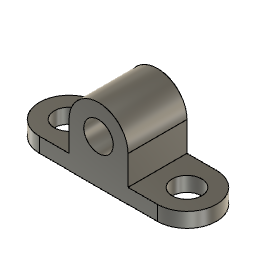
A4 v0 (Autodesk Fusion 360 design; units mm, degrees)
Autodesk Fusion 360 part; units mm, degrees
sketch "Sketch1" plane through (0, 0, 0) normal (0, 0, 1) x (1, 0, 0)
  line L0 (40, -20) -> (-40, -20)
  line L1 (-40, 20) -> (40, 20)
  circle A0 centre (40, 0) radius 10
  circle A1 centre (-40, 0) radius 10
  arc A2 (24, -12) -> (40, 20) centre (40, 0) ccw
  arc A3 (-40, 20) -> (-40, -20) centre (-40, 0) ccw
  dimension "d1" = 80
  dimension "d2" = 40
  dimension "d5" = 40
  dimension "d6" = 40
  constraint horizontal L0
  constraint parallel L0 L1
  measures "d1" distance of L1.start L1.end
  measures "d2" distance of L0.end L1.start
  measures "d5" diameter of A2
  measures "d6" diameter of A3
extrude "Extrude1" add sketch "Sketch1" along normal blind 10
sketch "Sketch2" plane through (0, 0, 0) normal (0, 1, 0) x (1, 0, 0)
  line L0 (-20, 0.1287) -> (20, 0.1287)
  line L1 (20, 0.1287) -> (20, -29.8713)
  line L2 (-20, -29.8713) -> (-20, 0.1287)
  line L3 (-40, 0) -> (-40, -10)
  circle A0 centre (0, -29.8713) radius 10
  arc A1 (-20, -29.8713) -> (20, -29.8713) centre (0, -29.8713) ccw
  dimension "d12" = 40
  dimension "d13" = 30
  dimension "d14" = 20
  dimension "d15" = 20
  dimension "d16" = 20
  constraint horizontal L0
  constraint vertical L1
  constraint vertical L2
  constraint concentric A0 A1
  measures "d12" distance of L0.start L0.end
  measures "d13" distance of L0.start L2.start
  measures "d14" distance of L2 L3
  measures "d15" radius of A1
  measures "d16" diameter of A0
extrude "Extrude2" add sketch "Sketch2" along normal mid plane 40
